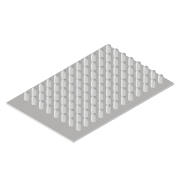
# Autodesk Inventor part: 00_96_LED_IR_PCB
Saved by Autodesk Inventor 2022.5 (Build 265521000, 521)
## iProperties
Created: 2023-11-03
Part Number: 00_96_LED_IR_PCB
Material: Generisch
Document SubType Name: Modeling
Designer: diederichbenedict
Density: 1 g/cm^3
Appearance: Vorgabe
Author: diederichbenedict
Autodesk Inventor part; units mm, degrees
ref_plane "YZ Plane" through (0, 0, 0) normal (1, 0, 0) x (0, 1, 0)
ref_plane "XZ Plane" through (0, 0, 0) normal (0, 1, 0) x (-1, 0, 0)
ref_plane "XY Plane" through (0, 0, 0) normal (0, 0, 1) x (1, 0, 0)
sketch "Skizze1" plane through (0, 0, 0) normal (0, 1, 0) x (-1, 0, 0)
  line L0 (-36, -54.25) -> (36, -54.25)
  line L1 (36, -54.25) -> (36, 54.25)
  line L2 (36, 54.25) -> (-36, 54.25)
  line L3 (-36, 54.25) -> (-36, -54.25)
  line L4 (-36, -54.25) -> (36, 54.25) construction
  line L5 (36, -54.25) -> (-36, 54.25) construction
  point P0 (0, 0)
  dimension "d0" = 72
  dimension "d1" = 108.5
  constraints: 12 end point, 2 midpoint, 2 parallel, 1 horizontal, 1 perpendicular
  measures "d0" distance of L2.end L1.end
  measures "d1" distance of L1.end L0.end
extrude "Extrusion1" add sketch "Skizze1" along normal blind 1.6
sketch "Skizze2" plane through (0, 1.6, 0) normal (0, 1, 0) x (1, 0, 0)
  circle A0 centre (-3.9832, 0) radius 2
  point P0 (0, 0)
  dimension "d4" = 4
  constraints: 1 centre point
  measures "d4" diameter of A0
extrude "Extrusion2" add sketch "Skizze2" along normal blind 7
fillet "Rundung1" radius 2 1 edges at (-5.9832, 8.6, 0)
pattern_linear "Rechteckige Anordnung1" count 8 spacing 8 along (1, 0, 0) count 12 spacing 8 along (0, 0, -1) of "Extrusion2", "Rundung1" first direction both ways yes second direction both ways yes
ref_plane "Arbeitsebene1" through (0, 0, 54.25) normal (1, 0, 0) x (0, 0, -1)
ref_plane "Arbeitsebene2" through (36, 0, 0) normal (0, 0, -1) x (-1, 0, 0)
